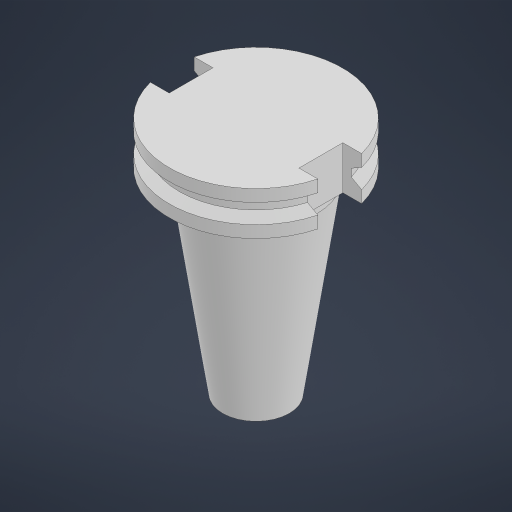
# Autodesk Inventor part: SK40Collar
Saved by Autodesk Inventor 2024.1 (Build 281209000, 209)
## iProperties
Created: 2023-12-31
Part Number: SK40Collar
Material: Generic
Document SubType Name: Modeling
Designer: fablabadmin
Density: 1 g/cm^3
Appearance: Default
Author: fablabadmin
Autodesk Inventor part; units mm, degrees
ref_plane "YZ Plane" through (0, 0, 0) normal (1, 0, 0) x (0, 1, 0)
ref_plane "XZ Plane" through (0, 0, 0) normal (0, 1, 0) x (-1, 0, 0)
ref_plane "XY Plane" through (0, 0, 0) normal (0, 0, 1) x (1, 0, 0)
sketch "Sketch1" plane through (0, 0, 0) normal (0, 0, 1) x (1, 0, 0)
  line L0 (-43.38, 0) -> (7.23, 0) construction
  line L1 (0, -97.41) -> (0, 25.51) projected
  line L2 (0, 7.95) -> (-31.775, 7.95)
  line L3 (-31.775, 7.95) -> (-31.775, 3.5363)
  line L4 (-31.775, 3.5363) -> (-28.125, 1.4289)
  line L5 (-28.125, 1.4289) -> (-28.125, -1.4289)
  line L6 (-31.775, -7.95) -> (0, -7.95)
  line L7 (-28.125, -1.4289) -> (-31.775, -3.5363)
  line L8 (-31.775, -3.5363) -> (-31.775, -7.95)
  circle A0 centre (-32.65, 0) radius 3.5 construction
  line L9 (-22.225, -7.95) -> (-22.225, -11.45)
  line L10 (-22.225, -11.45) -> (0, -11.45) construction
  line L11 (-22.225, -11.45) -> (-12.2465, -79.85)
  line L12 (-12.2465, -79.85) -> (-8, -79.85)
  line L13 (-8, -79.85) -> (-8, -54.85)
  line L14 (-8, -54.85) -> (0, -54.85)
  point P0 (0, 0)
  point P1 (-36.15, 0)
  dimension "d5" = 7
  dimension "d0" = 60
  dimension "d1" = 56.25
  dimension "d2" = 63.55
  dimension "d3" = 15.9
  dimension "d6" = 72.3
  dimension "d14" = 3.5
  dimension "d15" = 44.45
  dimension "d16" = 68.4
  dimension "d17" = 8.3
  dimension "d18" = 25
  dimension "d19" = 16
  dimension "d20" = 24.493
  constraints: 26 end point, 7 point on line, 5 perpendicular, 2 equal length, 2 horizontal, 2 vertical, 1 horizontal alignment, 1 parallel, 1 symmetric about line, 4 other
  measures "d0" angle of L7 L4
  measures "d1" diameter of L5 L1
  measures "d2" diameter of L3 L1
  measures "d3" distance between parallel lines of L6 L2
  measures "d6" diameter of point (-36.15, 0) L1
  measures "d14" distance of L9.start L9.end
  measures "d15" diameter of L9 L1
  measures "d16" distance from line of L9.end L12
  measures "d17" angle of L1 L11
  measures "d18" distance of L12.end L13.end
  measures "d19" diameter of L13 L1
  measures "d20" diameter of L11.end L1
revolve "Revolution1" add sketch "Sketch1" angle 360 about axis through (0, -10, 0) along (0, 1, 0)
sketch "Sketch2" plane through (0, 7.95, 0) normal (0, 1, 0) x (1, 0, 0)
  circle A0 centre (0, 0) radius 31.775 construction
  line L0 (-44.485, 0) -> (44.485, 0) construction
  line L1 (0, 44.485) -> (0, -44.485) construction
  line L2 (-31.775, 8.05) -> (-23.825, 8.05)
  line L3 (-23.825, 8.05) -> (-23.825, -8.05)
  line L4 (-23.825, -8.05) -> (-31.775, -8.05)
  line L5 (-31.775, -8.05) -> (-31.775, 8.05)
  circle A1 centre (0, 0) radius 31.775 projected
  line L6 (31.775, 8.05) -> (23.825, 8.05)
  line L7 (23.825, 8.05) -> (23.825, -8.05)
  line L8 (23.825, -8.05) -> (31.775, -8.05)
  line L9 (31.775, -8.05) -> (31.775, 8.05)
  point P0 (-31.775, 0)
  point P1 (31.775, 0)
  point P2 (30.7384, -8.05)
  point P3 (30.7384, 8.05)
  point P4 (-30.7384, 8.05)
  point P5 (-30.7384, -8.05)
  dimension "d12" = 16.1
  dimension "d13" = 47.65
  constraints: 16 end point, 5 symmetric about line, 2 parallel, 1 horizontal, 1 midpoint, 1 perpendicular, 3 other
  measures "d12" distance of L4.end L2.start
  measures "d13" distance between parallel lines of L7 L3
extrude "Extrusion1" cut sketch "Sketch2" against normal through all contours L2 L3 L4 A1 | A1 L8 L7 L6
body "Solid1"
